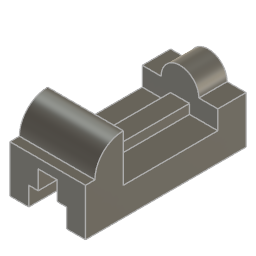
cad2 (Autodesk Fusion 360 design; units mm, degrees)
part number: 2026-02-27-05-21-05-320
Autodesk Fusion 360 part; units mm, degrees
sketch "Sketch1" plane through (0, 0, 0) normal (0, 1, 0) x (1, 0, 0)
  line L0 (0, 0) -> (0, -5)
  line L1 (0, -5) -> (8, -5)
  line L2 (8, -5) -> (8, 0)
  line L3 (8, 0) -> (6, 0)
  line L4 (6, 0) -> (6, -2)
  line L5 (6, -2) -> (5, -2)
  line L6 (5, -2) -> (5, -4)
  line L7 (5, -4) -> (3, -4)
  line L8 (3, -4) -> (3, -2)
  line L9 (3, -2) -> (2, -2)
  line L10 (2, -2) -> (2, 0)
  line L11 (2, 0) -> (0, 0)
  dimension "d1" = 8
  dimension "d2" = 2
  constraint coincident L0.start L11.end
  constraint vertical L0
  constraint perpendicular L0 L1
  constraint perpendicular L1 L2
  constraint perpendicular L2 L3
  constraint perpendicular L3 L4
  constraint perpendicular L4 L5
  constraint perpendicular L5 L6
  constraint perpendicular L6 L7
  constraint perpendicular L7 L8
  constraint perpendicular L6 L9
  constraint perpendicular L9 L10
  constraint perpendicular L0 L11
  measures "d1" distance of L0.end L1.end
  measures "d2" distance of L2.end L3.end
extrude "Extrude1" add sketch "Sketch1" along normal blind 1
sketch "Sketch2" plane through (8, 0, 0) normal (1, 0, 0) x (0, 1, 0)
  line L0 (0, 5) -> (0, 0)
  line L1 (0, 0) -> (1, 0)
  line L2 (1, 0) -> (1, 5)
  line L3 (1, 5) -> (0, 5)
  line L4 (1, 5) -> (4, 5)
  line L5 (4, 5) -> (4, 8)
  arc A0 (4, 8) -> (1, 5) centre (4, 5) ccw
  line L6 (4, 5) -> (4, 0)
  line L7 (4, 0) -> (1, 0)
  dimension "d5" = 3
  dimension "d6" = 3
  constraint coincident L2.end L3.start
  constraint perpendicular L2 L4
  constraint perpendicular L4 L5
  constraint coincident L4.end L5.start
  constraint perpendicular L4 L6
  constraint coincident L1.end L2.start
  constraint perpendicular L6 L7
  measures "d5" distance of L2.end L4.end
  measures "d6" distance of L4.end L5.end
extrude "Extrude2" add sketch "Sketch2" against normal blind 8 contours L2 L4 L6 L7 | L4 L5 A0
extrude "Extrude3" cut 1 faces at (4.3333, 1, 0.6667) along direction (0, 1, 0) blind 4.5
sketch "Sketch3" plane through (0, 4, 0) normal (0, 1, 0) x (-1, 0, 0)
  line L0 (-2, 2) -> (-2, 0)
  line L1 (-2, 0) -> (0, 0)
  line L2 (0, 0) -> (0, 8)
  line L3 (0, 8) -> (-8, 8)
  line L4 (-8, 8) -> (-8, 0)
  line L5 (-8, 0) -> (-6, 0)
  line L6 (-6, 0) -> (-6, 2)
  line L7 (-6, 2) -> (-5, 2)
  line L8 (-5, 2) -> (-5, 4)
  line L9 (-5, 4) -> (-3, 4)
  line L10 (-3, 4) -> (-3, 2)
  line L11 (-3, 2) -> (-2, 2)
  line L12 (-8, 0) -> (-8, 3)
  line L13 (-8, 3) -> (-5, 3)
  line L14 (-5, 3) -> (-5, 4)
  line L15 (-3, 4) -> (-3, 3)
  line L16 (-3, 3) -> (0, 3)
  line L17 (-3, 4) -> (-5, 4)
  line L18 (0, 3) -> (0, 0)
  line L19 (-8, 0) -> (0, 0)
  dimension "d11" = 3
  dimension "d12" = 3
  constraint coincident L4.end L5.start
  constraint perpendicular L5 L12
  constraint perpendicular L8 L13
  constraint coincident L8.end L9.start
  constraint coincident L9.end L10.start
  constraint midpoint L10 L15.end
  constraint coincident L2 L16.end
  constraint perpendicular L2 L16
  constraint coincident L1.end L2.start
  measures "d11" distance of L4.end L12.end
  measures "d12" distance of L12.end L13.end
extrude "Extrude4" add sketch "Sketch3" along normal blind 10 contours L0 L1 L2 L10 L11 L16 L18 L19 | L0 L6 L7 L8 L9 L10 L11 L14 L15 L17 L19 | L4 L5 L6 L7 L8 L12 L13 L19
sketch "Sketch4" plane through (0, 14, 0) normal (0, 1, 0) x (-1, 0, 0)
  line L0 (-8, 3) -> (-8, 0)
  line L1 (-8, 0) -> (0, 0)
  line L2 (0, 0) -> (0, 3)
  line L3 (0, 3) -> (-3, 3)
  line L4 (-3, 3) -> (-3, 4)
  line L5 (-3, 4) -> (-5, 4)
  line L6 (-5, 4) -> (-5, 3)
  line L7 (-5, 3) -> (-8, 3)
  line L8 (-8, 0) -> (-8, 5)
  line L9 (-8, 5) -> (-6, 5)
  line L10 (-6, 5) -> (-4, 5)
  arc A0 (-2, 5) -> (-6, 5) centre (-4, 5) ccw
  line L11 (-2, 5) -> (0, 5)
  line L12 (0, 5) -> (0, 0)
  dimension "d15" = 5
  dimension "d16" = 2
  constraint coincident L0.end L1.start
  constraint perpendicular L1 L8
  constraint perpendicular L8 L9
  constraint perpendicular L8 L10
  constraint coincident L10.end A0.centre
  constraint horizontal L11
  constraint coincident L1.end L2.start
  constraint perpendicular L1 L12
  measures "d15" distance of L0.end L8.end
  measures "d16" distance of L8.end L9.end
extrude "Extrude5" add sketch "Sketch4" along normal blind 3
